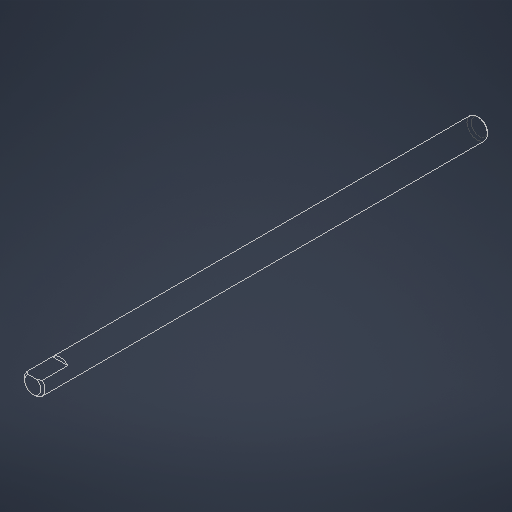
# Autodesk Inventor part: popychacz
Saved by Autodesk Inventor 2026.1 (Build 301233020, 233B)
## iProperties
Created: 2026-02-27
Part Number: popychacz
Material: Generic
Document SubType Name: Modeling
Designer: Jan
Density: 1 g/cm^3
Appearance: Default
Author: Jan
Autodesk Inventor part; units mm, degrees
ref_plane "YZ Plane" through (0, 0, 0) normal (1, 0, 0) x (0, 1, 0)
ref_plane "XZ Plane" through (0, 0, 0) normal (0, 1, 0) x (-1, 0, 0)
ref_plane "XY Plane" through (0, 0, 0) normal (0, 0, 1) x (1, 0, 0)
sketch "Sketch1" plane through (0, 0, 0) normal (0, 0, 1) x (1, 0, 0)
  circle A0 centre (0, 0) radius 3
  dimension "d0" = 6
  constraints: 1 centre point, 1 coincident
  measures "d0" diameter of A0
extrude "Extrusion1" add sketch "Sketch1" along normal blind 130
thread "Thread1" size "M6x0.5" class "6g" standard "ISO Metric profile" full length
chamfer "Chamfer1" distance 0.6 angle 45 1 edges at (-3, 0, 130)
chamfer "Chamfer2" distance 0.6 angle 45 1 edges at (-3, 0, 0)
sketch "Sketch2" plane through (0, 0, 130) normal (0, 0, 1) x (1, 0, 0)
  line L0 (3.8696, 4.6025) -> (-3.8038, 4.6025)
  line L1 (-3.8038, 4.6025) -> (-3.8038, 2)
  line L2 (-3.8038, 2) -> (3.8696, 2)
  line L3 (3.8696, 2) -> (3.8696, 4.6025)
  point P0 (0, 0)
  dimension "d11" = 2
  constraints: 8 end point, 2 parallel, 1 horizontal, 1 perpendicular
  measures "d11" distance from line of point (0, 0) L2
extrude "Extrusion2" cut sketch "Sketch2" against normal blind 8
body "Solid1"
